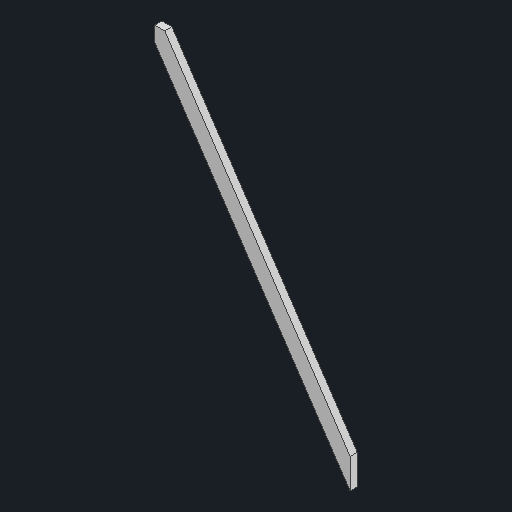
# Autodesk Inventor part: S_2x4x76.102
Saved by Autodesk Inventor 2026 (Build 300175000, 175)
## iProperties
Created: 2025-09-04
Part Number: S_2x4x76.102
Material: Generic
Document SubType Name: Modeling
Designer: trott
Density: 1 g/cm^3
Appearance: Default
Author: trott
Autodesk Inventor part; units mm, degrees
ref_plane "YZ Plane" through (0, 0, 0) normal (1, 0, 0) x (0, 1, 0)
ref_plane "XZ Plane" through (0, 0, 0) normal (0, 1, 0) x (-1, 0, 0)
ref_plane "XY Plane" through (0, 0, 0) normal (0, 0, 1) x (1, 0, 0)
sketch "Sketch1" plane through (0, 0, 0) normal (0, 0, 1) x (1, 0, 0)
  line L0 (-520.7, -1549.4) -> (520.7, -1549.4)
  line L1 (520.7, -1549.4) -> (520.7, 1549.4)
  line L2 (520.7, 1549.4) -> (-520.7, 1549.4)
  line L3 (-520.7, 1549.4) -> (-520.7, -1549.4)
  line L4 (-520.7, -1549.4) -> (520.7, 1549.4) construction
  line L5 (520.7, -1549.4) -> (-520.7, 1549.4) construction
  line L6 (-520.7, 0) -> (520.7, 0)
  line L7 (520.7, 0) -> (-520.7, -1549.4)
  line L8 (-483.8087, -1574.1958) -> (-557.5913, -1524.6042)
  line L9 (557.5913, -24.7958) -> (483.8087, 24.7958)
  line L10 (483.8087, 24.7958) -> (-557.5913, -1524.6042)
  line L11 (-483.8087, -1574.1958) -> (557.5913, -24.7958)
  line L12 (483.8087, 24.7958) -> (520.7, 79.6829)
  line L13 (-520.7, 1549.4) -> (520.7, -1549.4) construction
  line L14 (520.7, 0) -> (-520.7, 1549.4)
  line L15 (-483.8087, 1574.1958) -> (-557.5913, 1524.6042)
  line L16 (557.5913, 24.7958) -> (483.8087, -24.7958)
  line L17 (483.8087, -24.7958) -> (-557.5913, 1524.6042)
  line L18 (-483.8087, 1574.1958) -> (557.5913, 24.7958)
  line L19 (483.8087, -24.7958) -> (520.7, -79.6829)
  point P0 (0, 0)
  point P1 (520.7, 79.6829)
  point P2 (-467.1426, 1549.4)
  point P3 (-520.7, 1469.7171)
  point P4 (520.7, -79.6829)
  point P5 (520.7, -79.6829)
  point P6 (467.1426, 0)
  point P7 (-520.7, -1469.7171)
  point P8 (-467.1426, -1549.4)
  dimension "d0" = 1041.4
  dimension "d1" = 3098.8
  dimension "d3" = 88.9
  dimension "d4" = 88.9
  constraints: 40 end point, 6 midpoint, 5 symmetric about line, 3 perpendicular, 3 point on line, 2 parallel, 1 horizontal
  measures "d0" distance of L2.end L1.end
  measures "d1" distance of L0.end L1.end
  measures "d3" distance of L8.start L8.end
  measures "d4" distance of L9.start L9.end
extrude "Extrusion1" add sketch "Sketch1" along normal blind 38.1 contours L19 L16 L7 | L7 L1 L19 | L10 L9 L6 | L17 L3 L14 L12 L10 | L6 L16 L17 | L14 L12 L1 | L9 L12 L14 | L12 L14 L2 L18
body "Solid1"
